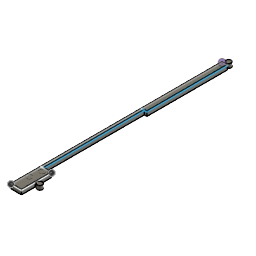
finger joint box (Autodesk Fusion 360 design; units mm, degrees)
part number: 2026-07-23-17-33-07-436
Autodesk Fusion 360 part; units mm, degrees
note: some values were not read from the file. Set by a fixed rule: which sketch regions a step uses.
pattern_linear "R-Pattern1" [no effect]
pattern_linear "R-Pattern2" [no effect]
pattern_linear "R-Pattern3" [no effect]
sketch "Sketch12" plane through (0, 0, 0) normal (0, 1, 0) x (1, 0, 0)
  line L0 (0, 0) -> (1.3, 0)
  line L1 (1.3, 0) -> (1.3, -90)
  line L2 (1.3, -90) -> (0, -90)
  line L3 (0, -90) -> (0, 0)
  line L4 (1.3, 0) -> (2.6, 0)
  line L5 (2.6, 0) -> (2.6, -40)
  line L6 (2.6, -40) -> (1.3, -40)
  line L7 (1.3, -40) -> (1.3, 0)
  line L8 (0, -90) -> (5.2, -90)
  line L9 (5.2, -90) -> (5.2, -105)
  line L10 (5.2, -105) -> (0, -105)
  line L11 (0, -105) -> (0, -90)
  line L12 (5.2, -90) -> (3.1568, -90)
  line L13 (3.1568, -90) -> (3.1568, -97.5)
  line L14 (3.1568, -97.5) -> (5.2, -97.5)
  line L15 (5.2, -97.5) -> (5.2, -90)
  line L16 (5.2, -97.5) -> (4.2, -97.5)
  line L17 (4.2, -97.5) -> (4.2, -98.15)
  line L18 (4.2, -98.15) -> (5.2, -98.15)
  line L19 (5.2, -98.15) -> (5.2, -97.5)
  line L20 (5.2, -98.15) -> (6.2, -98.15)
  line L21 (6.2, -98.15) -> (6.2, -96.85)
  line L22 (6.2, -96.85) -> (5.2, -96.85)
  line L23 (5.2, -96.85) -> (5.2, -98.15)
  line L24 (6.2, -96.85) -> (6.85, -96.85)
  line L25 (6.85, -96.85) -> (6.85, -97.5)
  line L26 (6.85, -97.5) -> (6.2, -97.5)
  line L27 (6.2, -97.5) -> (6.2, -96.85)
  circle A0 centre (6.85, -97.5) radius 1.3
  line L28 (5.2, -97.5) -> (0, -97.5)
  line L29 (0, -97.5) -> (0, -98.15)
  line L30 (0, -98.15) -> (5.2, -98.15)
  line L31 (5.2, -98.15) -> (5.2, -97.5)
  line L32 (0, -98.15) -> (1.65, -98.15)
  line L33 (1.65, -98.15) -> (1.65, -96.85)
  line L34 (1.65, -96.85) -> (0, -96.85)
  line L35 (0, -96.85) -> (0, -98.15)
  circle A1 centre (1.65, -97.5) radius 1.37
  line L36 (0, -97.5) -> (1, -97.5)
  line L37 (1, -97.5) -> (1, -96.78)
  line L38 (1, -96.78) -> (0, -96.78)
  line L39 (0, -96.78) -> (0, -97.5)
  line L40 (0, -97.5) -> (1, -97.5)
  line L41 (1, -97.5) -> (1, -98.22)
  line L42 (1, -98.22) -> (0, -98.22)
  line L43 (0, -98.22) -> (0, -97.5)
  line L44 (1.3, -90) -> (2.6, -90)
  line L45 (2.6, -90) -> (3.1, -90)
  line L46 (3.1, -90) -> (1.8, -90)
  line L47 (1.3, 0) -> (0.65, 0)
  line L48 (0.65, 0) -> (0.65, -0.65)
  line L49 (0.65, -0.65) -> (1.3, -0.65)
  line L50 (1.3, -0.65) -> (1.3, 0)
  line L51 (0.65, 0) -> (1.95, 0)
  line L52 (1.95, 0) -> (1.95, 1.95)
  line L53 (1.95, 1.95) -> (0.65, 1.95)
  line L54 (0.65, 1.95) -> (0.65, 0)
  circle A2 centre (1.3, 1.95) radius 1.3
  line L55 (1.3, -90) -> (3.9, -90)
  line L56 (3.9, -90) -> (3.9, -92.6)
  line L57 (3.9, -92.6) -> (1.3, -92.6)
  line L58 (1.3, -92.6) -> (1.3, -90)
  line L59 (2.6, -90) -> (3.32, -90)
  line L60 (3.32, -90) -> (3.32, -91.3)
  line L61 (3.32, -91.3) -> (2.6, -91.3)
  line L62 (2.6, -91.3) -> (2.6, -90)
  line L63 (2.6, -90) -> (1.88, -90)
  line L64 (1.88, -90) -> (1.88, -91.95)
  line L65 (1.88, -91.95) -> (2.6, -91.95)
  line L66 (2.6, -91.95) -> (2.6, -90)
  circle A3 centre (2.6, -91.95) radius 1.37
  dimension "d59" = 1.3
  dimension "d60" = 90
  dimension "d62" = 1.3
  dimension "d63" = 40
  dimension "d64" = 5.2
  dimension "d65" = 15
  dimension "d66" = 7.5
  dimension "d67" = 1
  dimension "d68" = 0.65
  dimension "d69" = 1
  dimension "d70" = 1.3
  dimension "d71" = 0.65
  dimension "d72" = 0.65
  dimension "d73" = 2.6
  dimension "d74" = 0.65
  dimension "d75" = 1.65
  dimension "d76" = 1.3
  dimension "d77" = 2.74
  dimension "d82" = 1
  dimension "d83" = 0.72
  dimension "d84" = 1
  dimension "d85" = 0.72
  dimension "d95" = 1.3
  dimension "d98" = 0.65
  dimension "d99" = 0.65
  dimension "d100" = 1.3
  dimension "d101" = 1.95
  dimension "d102" = 2.6
  dimension "d106" = 2.6
  dimension "d107" = 2.6
  dimension "d108" = 0.72
  dimension "d109" = 1.3
  dimension "d110" = 0.72
  dimension "d111" = 1.95
  dimension "d119" = 2.74
  constraint horizontal L0
  constraint vertical L1
  constraint horizontal L2
  constraint vertical L3
  constraint coincident L0.start L3.end
  constraint horizontal L4
  constraint vertical L5
  constraint horizontal L6
  constraint vertical L7
  constraint horizontal L8
  constraint vertical L9
  constraint horizontal L10
  constraint vertical L11
  constraint horizontal L12
  constraint vertical L13
  constraint horizontal L14
  constraint vertical L15
  constraint horizontal L16
  constraint vertical L17
  constraint horizontal L18
  constraint vertical L19
  constraint horizontal L20
  constraint vertical L21
  constraint horizontal L22
  constraint vertical L23
  constraint horizontal L24
  constraint vertical L25
  constraint horizontal L26
  constraint vertical L27
  constraint coincident L25.end L26.start
  constraint horizontal L28
  constraint vertical L29
  constraint horizontal L30
  constraint vertical L31
  constraint horizontal L32
  constraint vertical L33
  constraint horizontal L34
  constraint vertical L35
  constraint midpoint L33 A1.centre
  constraint horizontal L36
  constraint vertical L37
  constraint horizontal L38
  constraint vertical L39
  constraint horizontal L40
  constraint vertical L41
  constraint horizontal L42
  constraint vertical L43
  constraint horizontal L44
  constraint horizontal L45
  constraint horizontal L46
  constraint horizontal L47
  constraint vertical L48
  constraint horizontal L49
  constraint vertical L50
  constraint horizontal L51
  constraint vertical L52
  constraint horizontal L53
  constraint vertical L54
  constraint midpoint L53 A2.centre
  constraint horizontal L55
  constraint vertical L56
  constraint horizontal L57
  constraint vertical L58
  constraint horizontal L59
  constraint vertical L60
  constraint horizontal L61
  constraint vertical L62
  constraint horizontal L63
  constraint vertical L64
  constraint horizontal L65
  constraint vertical L66
  constraint coincident L65.end L66.start
  measures "d59" distance of L0.start L0.end
  measures "d60" distance of L0.start L2.end
  measures "d62" distance of L0.end L4.end
  measures "d63" distance of L0.end L6.end
  measures "d64" distance of L2.end L8.end
  measures "d65" distance of L2.end L10.end
  measures "d66" distance of L8.end L14.end
  measures "d67" distance of L14.end L16.end
  measures "d68" distance of L14.end L18.end
  measures "d69" distance of L18.end L20.end
  measures "d70" distance of L18.end L22.end
  measures "d71" distance of L21.end L24.end
  measures "d72" distance of L21.end L26.end
  measures "d73" diameter of A0
  measures "d74" distance of L14.end L18.end
  measures "d75" distance of L29.end L32.end
  measures "d76" distance of L29.end L34.end
  measures "d77" diameter of A1
  measures "d82" distance of L28.end L36.end
  measures "d83" distance of L28.end L38.end
  measures "d84" distance of L28.end L36.end
  measures "d85" distance of L28.end L42.end
  measures "d95" distance of L45.end L46.end
  measures "d98" distance of L0.end L47.end
  measures "d99" distance of L0.end L49.end
  measures "d100" distance of L47.end L51.end
  measures "d101" distance of L47.end L53.end
  measures "d102" diameter of A2
  measures "d106" distance of L1.end L55.end
  measures "d107" distance of L1.end L57.end
  measures "d108" distance of L44.end L59.end
  measures "d109" distance of L44.end L61.end
  measures "d110" distance of L44.end L63.end
  measures "d111" distance of L44.end L65.end
  measures "d119" diameter of A3
other "Base Mesh Feature3"
sketch "Sketch15" plane through (0, 2, 0) normal (0, 1, 0) x (-1, 0, 0)
  line L0 (0, 90) -> (0, 96.78)
  line L1 (0, 96.78) -> (-0.4845, 96.78)
  arc A0 (-0.4845, 98.22) -> (-0.4845, 96.78) centre (-1.65, 97.5) ccw
  line L2 (-0.4845, 98.22) -> (0, 98.22)
  line L3 (0, 98.22) -> (0, 105)
  line L4 (0, 105) -> (-5.2, 105)
  line L5 (-5.2, 105) -> (-5.2, 90)
  line L6 (-5.2, 90) -> (0, 90)
  line L7 (0, 105) -> (-5.2, 105)
  line L8 (-5.2, 105) -> (-5.2, 90)
  line L9 (-5.2, 90) -> (0, 90)
  line L10 (0, 90) -> (0, 105)
  line L11 (0, 0) -> (-2.6, 0)
  line L12 (-2.6, 0) -> (-2.6, 40)
  line L13 (-2.6, 40) -> (0, 40)
  line L14 (0, 40) -> (0, 0)
  line L15 (0, 90) -> (-1.3, 90)
  line L16 (-1.3, 90) -> (-1.3, 40)
  line L17 (-1.3, 40) -> (0, 40)
  line L18 (0, 40) -> (0, 90)
  constraint horizontal L7
  constraint vertical L8
  constraint horizontal L9
  constraint vertical L10
  constraint coincident L5.end L6.start
  constraint coincident L3.end L4.start
  constraint horizontal L11
  constraint vertical L12
  constraint horizontal L13
  constraint vertical L14
  constraint coincident L11.start L14.end
  constraint horizontal L15
  constraint vertical L16
  constraint horizontal L17
  constraint vertical L18
extrude "Extrude16" add sketch "Sketch12" along normal blind 2 contours L0 L1 L2 L3 L7 L8 L48 L49 | L0 L4 L47 L51 L52 L54 A2 | L0 L1 L7 L47 L48 L49 L50 L51 | L2 L8 L11 L13 L28 A1 L38 L57 L58 A3 | L1 L4 L5 L6 L7 L50 L51 | L52 L53 L54 A2 | L52 L53 L54 A2 | L8 L44 L46 L55 L58 L64 A3 | L14 L17 L28 L30 A1 | L8 L9 L12 L13 L14 L15 L16 L23 L28 L56 L57 A3 | L9 L10 L11 L18 L30 A1 L42 | L9 L14 L16 L17 L18 L19 L23 L28 L30 L31 | L8 L12 L55 L56 L60 A3 | L9 L15 L19 L20 L22 L23 A0 L31 | L20 L21 L22 L27 A0 | L20 L21 L22 L24 L25 L26 A0 | L21 L24 L25 L26 L27
extrude "Extrude17" add sketch "Sketch15" along normal blind 0.4
equation "length = 1100 mm"
equation "width = 700 mm"
equation "height = 500 mm"
equation "thickness = 18 mm"
equation "lengthFingers = 5"
equation "widthFingers = 3"
equation "heightFingers = 2"
equation "lengthFingersWidth = length / ( ( lengthFingers * 2 ) + 1 )"
equation "widthFingersWidth = width / ( ( widthFingers * 2 ) + 1 )"
equation "heightFingersWidth = height / ( ( heightFingers * 2 ) + 1 )"
equation "d20 = lengthFingers"
equation "d22 = length - ( lengthFingersWidth * 3 )"
equation "d32 = heightFingers"
equation "d34 = height - ( heightFingersWidth * 3 )"
equation "d45 = widthFingers"
equation "d47 = -( width - widthFingersWidth * 3 )"
equation "strip_width = 1.3 mm"
equation "strip_length = 90 mm"
equation "strip_depth = 2 mm"
equation "strip_support_width = 15 mm"
equation "d59 = strip_width"
equation "d60 = strip_length"
equation "strip_hole_length = 10 mm"
equation "d62 = strip_width"
equation "d63 = ( strip_length - strip_hole_length ) / 2"
equation "d64 = strip_width * 4"
equation "d65 = strip_support_width"
equation "d66 = strip_support_width / 2"
equation "d68 = strip_width / 2"
equation "d70 = strip_width"
equation "d71 = strip_width / 2"
equation "d72 = strip_width / 2"
equation "d73 = strip_width * 2"
equation "d74 = strip_width / 2"
equation "d75 = 1 mm + ( strip_width / 2 )"
equation "d76 = strip_width"
equation "d77 = ( strip_width * 2 ) + ( strip_clip_play * 2 )"
equation "strip_clip_width = 1.3 mm"
equation "strip_clip_play = 0.07 mm"
equation "d83 = strip_width / 2 + ( strip_clip_play )"
equation "d85 = strip_width / 2 + ( strip_clip_play )"
equation "strip_support_wall = 0.4 mm"
equation "d95 = strip_clip_width"
equation "d98 = strip_clip_width / 2"
equation "d99 = strip_clip_width / 2"
equation "d100 = strip_clip_width"
equation "d101 = strip_clip_width * 1.5"
equation "d102 = strip_clip_width * 2"
equation "d106 = strip_width * 2"
equation "d107 = strip_width * 2"
equation "d108 = ( strip_clip_width / 2 ) + ( strip_clip_play )"
equation "d109 = strip_clip_width"
equation "d110 = ( strip_clip_width / 2 ) + ( strip_clip_play )"
equation "d111 = strip_clip_width * 1.5"
equation "d119 = strip_clip_width * 2 + ( 2 * strip_clip_play )"
equation "d120 = strip_depth"
equation "d122 = strip_support_wall"
